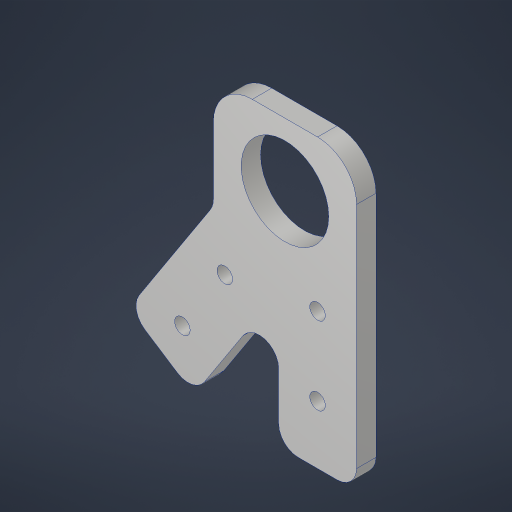
# Autodesk Inventor part: CL4-010
Saved by Autodesk Inventor 2023.4 (Build 274418000, 418)
## iProperties
Created: 2025-02-04
Part Number: CL4-010
Material: Aluminum 6061
Document SubType Name: Modeling
Designer: brand
Density: 2.7 g/cm^3
Appearance: Aluminum - Flat
Author: brand
Autodesk Inventor part; units mm, degrees
ref_plane "YZ Plane" through (0, 0, 0) normal (1, 0, 0) x (0, 1, 0)
ref_plane "XZ Plane" through (0, 0, 0) normal (0, 1, 0) x (-1, 0, 0)
ref_plane "XY Plane" through (0, 0, 0) normal (0, 0, 1) x (1, 0, 0)
sketch "Sketch1" plane through (0, 0, 0) normal (0, 0, 1) x (1, 0, 0)
  line L0 (-12.7, 0) -> (12.7, 0) construction
  line L1 (12.7, 0) -> (12.7, -57.15)
  line L2 (12.7, -57.15) -> (-12.7, -57.15)
  line L3 (-12.7, -57.15) -> (-12.7, 0) construction
  line L4 (-34.0022, 0) -> (-12.7, -13.8338) construction
  line L5 (-12.7, -13.8338) -> (-40.3677, -56.4383)
  line L6 (-40.3677, -56.4383) -> (-61.6699, -42.6045)
  line L7 (-61.6699, -42.6045) -> (-34.0022, 0)
  line L8 (-23.3511, -6.9169) -> (-51.0188, -49.5214) construction
  line L9 (-34.0022, 0) -> (12.7, 0)
  line L10 (-12.7, -13.8338) -> (-12.7, -57.15)
  point P0 (0, 0)
  point P1 (0, 0)
  point P2 (-30.268, -17.568)
  point P3 (-44.1019, -38.8703)
  point P4 (0, -12.7)
  point P5 (0, -38.1)
  dimension "d0" = 25.4
  dimension "d1" = 25.4
  dimension "d2" = 33
  dimension "d3" = 50.8
  dimension "d4" = 25.4
  dimension "d5" = 12.7
  dimension "d6" = 25.4
  dimension "d7" = 12.7
  dimension "d8" = 57.15
  constraints: 22 end point, 4 perpendicular, 3 midpoint, 3 parallel, 3 point on line, 2 horizontal, 2 vertical alignment, 1 coincident, 1 horizontal alignment, 1 vertical
  measures "d0" distance of L1.end L2.end
  measures "d1" distance of L4.start L4.end
  measures "d2" angle of L3 L5
  measures "d3" distance of L8.start L8.end
  measures "d4" distance of point (-44.102, -38.87) point (-30.268, -17.568)
  measures "d5" distance from line of L4 point (-30.268, -17.568)
  measures "d6" distance of point (0, -38.1) point (0, -12.7)
  measures "d7" distance of point (0, 0) point (0, -12.7)
  measures "d8" distance of L0.end L1.end
extrude "Extrusion1" add sketch "Sketch1" against normal blind 6.35
hole "Hole1" at (-30.268, -17.568, 0) at (-44.1019, -38.8703, 0) at (0, -12.7, 0) at (0, -38.1, 0) direction (0, 0, -1) diameter 5.1054 end through all clearance for "Flat Head Machine Screw (82)" size "#10" standard "Ansi Unified Screw Threads"
sketch "Sketch2" plane through (0, 0, 0) normal (0, 0, 1) x (1, 0, 0)
  circle A0 centre (0, -12.7) radius 2.5527 construction
  circle A1 centre (-30.268, -17.568) radius 2.5527 construction
  circle A2 centre (-44.1019, -38.8703) radius 2.5527 construction
  circle A3 centre (0, -38.1) radius 2.5527 construction
  line L0 (-12.7, -57.15) -> (12.7, -57.15) construction
  line L1 (12.7, -57.15) -> (12.7, 0) construction
  line L2 (12.7, 0) -> (-34.0022, 0) projected
  line L3 (-34.0022, 0) -> (-61.6699, -42.6045) construction
  line L4 (-61.6699, -42.6045) -> (-40.3677, -56.4383) construction
  line L5 (-40.3677, -56.4383) -> (-12.7, -13.8338) construction
  line L6 (-12.7, -13.8338) -> (-12.7, -57.15) construction
  circle A4 centre (0, -12.7) radius 2.5527 construction
  circle A5 centre (-30.268, -17.568) radius 2.5527 construction
  circle A6 centre (-44.1019, -38.8703) radius 2.5527 construction
  circle A7 centre (0, -38.1) radius 2.5527 construction
  line L7 (12.7, 0) -> (12.7, -57.15) construction
  line L8 (12.7, -57.15) -> (-12.7, -57.15) construction
  line L9 (-12.7, -57.15) -> (-12.7, -13.8338) construction
  line L10 (-12.7, -13.8338) -> (-40.3677, -56.4383) construction
  line L11 (-40.3677, -56.4383) -> (-61.6699, -42.6045) construction
  line L12 (-61.6699, -42.6045) -> (-34.0022, 0) construction
  line L13 (-34.0022, 0) -> (12.7, 0) construction
  circle A8 centre (-10.6511, 15.875) radius 14.2875 construction
  line L14 (12.7, 0) -> (-34.0022, 0) construction
  line L15 (-34.0022, 0) -> (-61.6699, -42.6045) construction
  circle A9 centre (0, -12.7) radius 2.5527 construction
  circle A10 centre (-30.268, -17.568) radius 2.5527 construction
  circle A11 centre (-44.1019, -38.8703) radius 2.5527 construction
  circle A12 centre (0, -38.1) radius 2.5527 construction
  line L16 (12.7, 0) -> (12.7, -57.15) construction
  line L17 (12.7, -57.15) -> (-12.7, -57.15) construction
  line L18 (-12.7, -57.15) -> (-12.7, -13.8338) construction
  line L19 (-12.7, -13.8338) -> (-40.3677, -56.4383) construction
  line L20 (-40.3677, -56.4383) -> (-61.6699, -42.6045) construction
  line L21 (-61.6699, -42.6045) -> (-34.0022, 0) construction
  line L22 (-34.0022, 0) -> (12.7, 0) construction
  line L23 (-34.0022, 0) -> (12.7, 0) construction
  line L24 (12.7, 0) -> (12.7, 36.5125)
  line L25 (12.7, 36.5125) -> (-34.0022, 36.5125)
  line L26 (-34.0022, 36.5125) -> (-34.0022, 0)
  point P0 (0, 0)
  point P1 (-10.6511, 0)
  point P2 (-10.6511, 0)
  point P3 (-10.6511, 30.1625)
  point P4 (-10.6511, 36.5125)
  dimension "d19" = 28.575
  dimension "d20" = 15.875
  dimension "d21" = 6.35
  constraints: 8 end point, 3 midpoint, 3 vertical alignment, 2 parallel, 1 coincident, 1 horizontal, 1 perpendicular, 2 other
  measures "d20" distance from line of L2 point (-10.651, 15.875)
  measures "d21" distance of point (-10.651, 36.513) point (-10.651, 30.163)
extrude "Extrusion2" add sketch "Sketch2" against normal up to surface (6.35 mm away)
hole "Hole2" at (-10.6511, 15.875, 0) direction (0, 0, -1) diameter 28.575 end through all
fillet "Fillet1" radius 6.35 6 edges at (12.7, -57.15, -3.175) (-12.7, -57.15, -3.175) (-12.7, -13.8338, -3.175) (-40.3677, -56.4383, -3.175) (-61.6699, -42.6045, -3.175) (-34.0022, 0, -3.175)
fillet "Fillet2" radius 12.7 2 edges at (-34.0022, 36.5125, -3.175) (12.7, 36.5125, -3.175)
body "Solid1"
